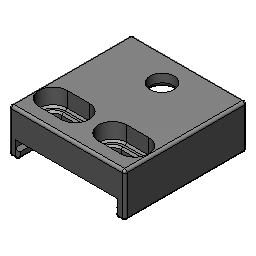
cam mount (Autodesk Fusion 360 design; units mm, degrees)
Autodesk Fusion 360 part; units mm, degrees
sketch "Sketch1" plane through (0, 0, 0) normal (0, 0, 1) x (1, 0, 0)
  line L0 (15, 16) -> (-15, 16)
  line L1 (-15, 16) -> (-15, -20)
  line L2 (-15, -20) -> (15, -20)
  line L3 (15, -20) -> (15, 16)
  line L4 (-15, 16) -> (-17, 16)
  line L5 (-17, 16) -> (-17, -20)
  line L6 (-17, -20) -> (-15, -20)
  line L7 (-15, -20) -> (-15, 16)
  line L8 (15, 16) -> (17, 16)
  line L9 (17, 16) -> (17, -20)
  line L10 (17, -20) -> (15, -20)
  line L11 (15, -20) -> (15, 16)
  circle A0 centre (0, 8) radius 3.5
  line L12 (-15, -12) -> (15, -12)
  circle A1 centre (5.5, -12) radius 2.5
  circle A2 centre (12, -12) radius 2.5
  line L13 (5.4997, -14.5) -> (12, -14.5)
  line L14 (11.9992, -9.5) -> (5.5, -9.5)
  line L15 (-15, -6) -> (15, -6)
  line L16 (17, -6) -> (15, -6)
  line L17 (-15, -6) -> (-17, -6)
  circle A3 centre (5.5, -12) radius 4.125
  circle A4 centre (12, -12) radius 4.125
  line L18 (5.5, -7.875) -> (12, -7.875)
  line L19 (5.5, -16.125) -> (12, -16.125)
  line L20 (0, 2.5) -> (0, 20)
  circle A5 centre (-5.5, -12) radius 4.125
  line L21 (-5.5, -16.125) -> (-12, -16.125)
  circle A6 centre (-5.5, -12) radius 2.5
  line L22 (-5.4997, -14.5) -> (-12, -14.5)
  line L23 (-11.9992, -9.5) -> (-5.5, -9.5)
  circle A7 centre (-12, -12) radius 4.125
  circle A8 centre (-12, -12) radius 2.5
  line L24 (-5.5, -7.875) -> (-12, -7.875)
  dimension "d1" = 30
  dimension "d3" = 2
  dimension "d4" = 7
  dimension "d12" = 6
  dimension "d13" = 8
  dimension "d28" = 5
  dimension "d29" = 2
  dimension "d45" = 20
  dimension "d46" = 16
  dimension "d49" = 8.25
  dimension "d50" = 8.25
  dimension "d51" = 3
  dimension "d52" = 15
  dimension "d53" = 6.5
  constraint horizontal L0
  constraint perpendicular L0 L1
  constraint parallel L0 L2
  constraint parallel L1 L3
  constraint horizontal L4
  constraint vertical L5
  constraint horizontal L6
  constraint vertical L7
  constraint horizontal L8
  constraint vertical L9
  constraint horizontal L10
  constraint vertical L11
  constraint coincident L7 L12.start
  constraint coincident L3 L12.end
  constraint perpendicular L3 L12
  constraint coincident L12 A1.centre
  constraint coincident L12 A2.centre
  constraint coincident A1 L13.start
  constraint coincident A2 L13.end
  constraint tangent A2 L13
  constraint coincident A2 L14.start
  constraint coincident A1 L14.end
  constraint tangent A1 L14
  constraint parallel L12 L14
  constraint coincident L7 L15.start
  constraint coincident L11 L15.end
  constraint perpendicular L11 L15
  constraint coincident L9 L16.start
  constraint perpendicular L3 L16
  constraint coincident L5 L17.end
  constraint perpendicular L5 L17
  constraint concentric A1 A3
  constraint concentric A2 A4
  constraint coincident A3 L18.start
  constraint coincident A4 L18.end
  constraint tangent A4 L18
  constraint tangent A3 L18
  constraint coincident A3 L19.start
  constraint coincident A4 L19.end
  constraint tangent A4 L19
  constraint tangent A3 L19
  constraint symmetric A1 L20 A6
  constraint symmetric A2 L20 A8
  constraint symmetric L13.start L20 L22.start
  constraint symmetric L13.end L20 L22.end
  constraint symmetric L14.start L20 L23.start
  constraint symmetric L14.end L20 L23.end
  constraint symmetric A3 L20 A5
  constraint symmetric A4 L20 A7
  constraint symmetric L19.start L20 L21.start
  constraint symmetric L19.end L20 L21.end
  constraint symmetric L18.start L20 L24.start
  constraint symmetric L18.end L20 L24.end
  measures "d1" distance of L1.end L2.end
  measures "d3" distance of L0.end L4.end
  measures "d4" diameter of A0
  measures "d12" distance of L12 L15
  measures "d13" distance of L2 L12
  measures "d28" diameter of A1
  measures "d29" distance of L0.start L8.end
  measures "d45" distance of L2 origin
  measures "d46" distance of origin L0
  measures "d49" diameter of A3
  measures "d50" diameter of A4
  measures "d51" distance of L11 A2.centre
  measures "d52" distance of origin L11
  measures "d53" distance of A2.centre A1.centre
extrude "Extrude1" add sketch "Sketch1" along normal blind 8 contours L0 L1 L3 L7 L11 L15 | L3 L8 L9 L11 L16 | L1 L4 L5 L7 L17
extrude "Extrude2" add sketch "Sketch1" along normal up to surface (8 mm away) contours L3 L9 L10 L11 L16 A4 | L1 L3 L7 L11 L12 L15 A3 A4 L18 A5 A7 L24 | L1 L5 L6 L7 L17 A7 | L1 L2 L3 L7 L11 L12 A3 A4 L19 A5 L21 A7
extrude "Extrude3" add sketch "Sketch1" against normal blind 5 contours L3 L8 L9 L11 L16 | L3 L9 L10 L11 L16 A4 | L1 L4 L5 L7 L17 | L3 L11 A4 | L1 L5 L6 L7 L17 A7 | L1 L7 A7
extrude "Extrude7" add sketch "Sketch1" along normal blind 3 contours L3 L11 A4 | L3 L11 L12 A2 L14 A3 A4 | L3 L11 L12 A2 L13 A3 A4 | A3 A4 L18 | L1 L7 L12 A5 L23 A7 A8 | L1 L7 A7 | L12 A1 L14 A3 A4 | L14 A3 A4 | L1 L7 L12 A5 L22 A7 A8 | A5 A7 L24 | A3 A4 L19 | L12 A1 L13 A3 A4 | A5 L23 A7 | L12 A5 A6 L23 A7 | A5 L21 A7 | L13 A3 A4 | L12 A5 A6 L22 A7 | A5 L22 A7
sketch "Sketch2" plane through (0, 0, 0) normal (0, 0, -1) x (1, 0, 0)
  circle A0 centre (0, -8) radius 3.5
  line L0 (15, -16) -> (15, 20)
  line L1 (15, 20) -> (-15, 20)
  line L2 (-15, 20) -> (-15, -16)
  line L3 (-15, -16) -> (15, -16)
  circle A1 centre (0, -8) radius 10
  arc A2 (5.4997, 14.5) -> (5.5, 9.5) centre (5.5, 12) ccw
  line L4 (5.4997, 14.5) -> (12, 14.5)
  arc A3 (11.9992, 9.5) -> (12, 14.5) centre (12, 12) ccw
  line L5 (11.9992, 9.5) -> (5.5, 9.5)
  arc A4 (-12, 14.5) -> (-11.9992, 9.5) centre (-12, 12) ccw
  line L6 (-12, 14.5) -> (-5.4997, 14.5)
  arc A5 (-5.5, 9.5) -> (-5.4997, 14.5) centre (-5.5, 12) ccw
  line L7 (-5.5, 9.5) -> (-11.9992, 9.5)
  dimension "d18" = 20
  constraint concentric A0 A1
  measures "d18" diameter of A1
extrude "Extrude4" cut sketch "Sketch2" against normal blind 4 contours L3 A1 | L3 A1
chamfer "Chamfer1" distance 4 distance2 20 2 edges at (-10.5, 16, 0) (10.5, 16, 0) measured on face at (12.6667, 16, 4) measured on face at (12.6667, 16, 4)
fillet "Fillet3" radius 1.5 1 edges at (-3.2631, 9.2657, 4)
chamfer "Chamfer3" distance 0.5 distance2 0.5 8 edges at (-8.7496, -9.5, 3) (-3, -11.9999, 3) (-8.7499, -14.5, 3) (-14.5, -11.9996, 3) (3, -11.9999, 3) (8.7496, -9.5, 3) (14.5, -11.9996, 3) (8.7499, -14.5, 3) measured on face at (-9.8331, -8.4167, 3) measured on face at (-9.8331, -8.4167, 3) measured on face at (-9.8331, -8.4167, 3) measured on face at (-9.8331, -8.4167, 3) measured on face at (9.8331, -8.4167, 3) measured on face at (9.8331, -8.4167, 3) measured on face at (9.8331, -8.4167, 3) measured on face at (9.8331, -8.4167, 3)
sketch "Sketch3" plane through (0, 16, 0) normal (0, 1, 0) x (-1, 0, 0)
  line L0 (15, 4) -> (15, -5)
  line L1 (15, -5) -> (17, -5)
  line L2 (17, -5) -> (17, 8)
  line L3 (17, 8) -> (-17, 8)
  line L4 (-17, 8) -> (-17, -5)
  line L5 (-17, -5) -> (-15, -5)
  line L6 (-15, -5) -> (-15, 4)
  line L7 (-15, 4) -> (-6, 4)
  line L8 (-15, -5) -> (-14.25, -5)
  line L9 (-14.25, -5) -> (-14.25, -3)
  line L10 (-14.25, -3) -> (-15, -3)
  line L11 (-15, -3) -> (-15, -5)
  line L12 (-15, -2) -> (-14.25, -3)
  line L13 (0, 20) -> (0, 2.5)
  line L14 (15, -2) -> (14.25, -3)
  line L15 (14.25, -5) -> (14.25, -3)
  line L16 (15, -5) -> (14.25, -5)
  line L17 (14.25, -3) -> (15, -3)
  line L18 (-6, 4) -> (6, 4)
  line L19 (6, 4) -> (15, 4)
  point P0 (15, 0)
  point P1 (-15, 0)
  dimension "d30" = 0.75
  dimension "d37" = 1
  dimension "d42" = 2
  dimension "d43" = 8
  constraint horizontal L8
  constraint vertical L9
  constraint horizontal L10
  constraint vertical L11
  constraint coincident L5.end L6.start
  constraint coincident L6 L12.start
  constraint symmetric L5.end L13 L0.end
  constraint symmetric L8.end L13 L15.start
  constraint symmetric L9.end L13 L14.end
  constraint symmetric L10.end L13 L17.end
  constraint symmetric L12.start L13 L14.start
  constraint coincident L0 P0
  constraint coincident L6 P1
  measures "d30" distance of L5.end L8.end
  measures "d37" distance of L10.end L12.start
  measures "d42" distance of L12.start P1
  measures "d43" distance of L3 P1
extrude "Extrude5" add sketch "Sketch3" against normal blind 5 contours L0 L14 L17 | L0 L15 L16 L17 | L6 L10 L12 | L6 L8 L9 L10 L11
sketch "Sketch4" plane through (0, -20, 0) normal (0, -1, 0) x (1, 0, 0)
  line L0 (-15, 0) -> (15, 0)
  line L1 (15, 0) -> (15, -5)
  line L2 (15, -5) -> (17, -5)
  line L3 (17, -5) -> (17, 8)
  line L4 (17, 8) -> (-17, 8)
  line L5 (-17, 8) -> (-17, -5)
  line L6 (-17, -5) -> (-15, -5)
  line L7 (-15, -5) -> (-15, 0)
  line L8 (15, -5) -> (14.25, -5)
  line L9 (14.25, -5) -> (14.25, -3)
  line L10 (14.25, -3) -> (15, -3)
  line L11 (15, -3) -> (15, -5)
  line L12 (14.25, -3) -> (15, -2)
  line L13 (0, 1.75) -> (0, 22.5)
  line L14 (-15, -5) -> (-14.25, -5)
  line L15 (-14.25, -5) -> (-14.25, -3)
  line L16 (-14.25, -3) -> (-15, -3)
  line L17 (-14.25, -3) -> (-15, -2)
  point P0 (15, 0)
  point P1 (-15, 0)
  dimension "d34" = 0.75
  dimension "d36" = 1
  dimension "d44" = 2
  constraint horizontal L8
  constraint vertical L9
  constraint horizontal L10
  constraint vertical L11
  constraint coincident L1.end L2.start
  constraint coincident L1 L12.end
  constraint symmetric L1.end L13 L6.end
  constraint symmetric L8.end L13 L14.end
  constraint symmetric L9.end L13 L15.end
  constraint symmetric L10.end L13 L16.end
  constraint symmetric L12.end L13 L17.end
  constraint coincident P0 L0.end
  constraint coincident L0.start L7.end
  measures "d34" distance of L1.end L8.end
  measures "d36" distance of L10.end L12.end
  measures "d44" distance of L12.end P0
extrude "Extrude6" add sketch "Sketch4" against normal blind 5 contours L7 L16 L17 | L1 L10 L12 | L7 L14 L15 L16 | L1 L8 L9 L10 L11
fillet "Fillet5" radius 0.75 4 edges at (-14.25, -17.5, -5) (-14.25, 13.5, -5) (14.25, -17.5, -5) (14.25, 13.5, -5)
fillet "Fillet6" radius 0.75 4 edges at (-17, -2, 8) (0, 16, 8) (17, -2, 8) (0, -20, 8)
fillet "Fillet7" radius 0.75 2 edges at (-17, -2, -5) (17, -2, -5)
fillet "Fillet8" radius 0.75 24 edges at (-14.25, -20, -3.625) (-14.4697, -20, -4.7803) (-15.625, -20, -5) (-16.7803, -20, -4.7803) (-17, -20, 1.5) (-16.7803, -19.7803, 7.7803) (14.25, -20, -3.625) (14.4697, -20, -4.7803) (15.625, -20, -5) (16.7803, -20, -4.7803) (17, -20, 1.5) (16.7803, -19.7803, 7.7803) (14.25, 16, -3.625) (14.4697, 16, -4.7803) (15.625, 16, -5) (16.7803, 16, -4.7803) (17, 16, 1.5) (16.7803, 15.7803, 7.7803) (-14.25, 16, -3.625) (-14.4697, 16, -4.7803) (-15.625, 16, -5) (-16.7803, 16, -4.7803) (-17, 16, 1.5) (-16.7803, 15.7803, 7.7803)
chamfer "Chamfer4" distance 0.5 angle 45 8 edges at (8.75, -7.875, 3) (16.125, -12, 3) (8.75, -16.125, 3) (1.375, -12, 3) (-8.75, -7.875, 3) (-1.375, -12, 3) (-8.75, -16.125, 3) (-16.125, -12, 3)
